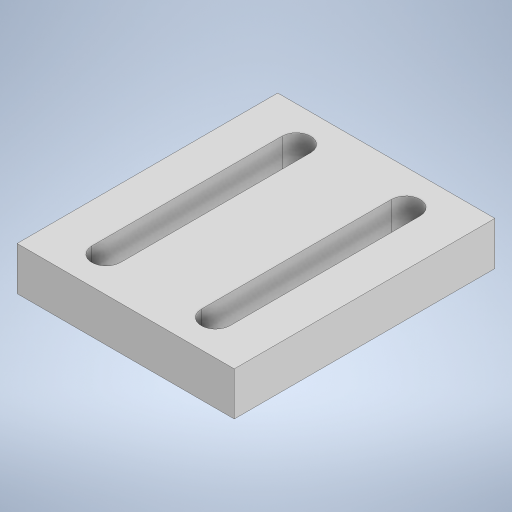
# Autodesk Inventor part: Fuß Steher
Saved by Autodesk Inventor 2024 (Build 280153000, 153)
## iProperties
Created: 2024-03-08
Part Number: Fuß Steher
Material: Generisch
Document SubType Name: Modeling
Designer: Andreas Weber
Density: 1 g/cm^3
Appearance: Vorgabe
Author: Andreas Weber
Autodesk Inventor part; units mm, degrees
ref_plane "YZ Plane" through (0, 0, 0) normal (1, 0, 0) x (0, 1, 0)
ref_plane "XZ Plane" through (0, 0, 0) normal (0, 1, 0) x (-1, 0, 0)
ref_plane "XY Plane" through (0, 0, 0) normal (0, 0, 1) x (1, 0, 0)
sketch "Skizze3" plane through (0, 0, 0) normal (0, 0, 1) x (1, 0, 0)
  line L0 (0, 0) -> (50, 0)
  line L1 (0, 0) -> (50, 0)
  line L2 (50, 0) -> (50, -60)
  line L3 (50, -60) -> (0, -60)
  line L4 (0, -60) -> (0, 0)
  line L5 (40.9, -4.8) -> (34.3, -4.8)
  line L6 (34.3, -4.8) -> (34.3, -55.2)
  line L7 (34.3, -55.2) -> (40.9, -55.2)
  line L8 (40.9, -55.2) -> (40.9, -4.8)
  line L9 (9.1, -4.8) -> (15.7, -4.8)
  line L10 (15.7, -4.8) -> (15.7, -55.2)
  line L11 (15.7, -55.2) -> (9.1, -55.2)
  line L12 (9.1, -55.2) -> (9.1, -4.8)
  dimension "d20" = 50
  dimension "d21" = 60
  dimension "d27" = 6.6
  dimension "d28" = 6.6
  constraints: 26 end point, 6 parallel, 4 horizontal, 3 perpendicular, 1 point on line
  measures "d20" distance of L2.end L3.end
  measures "d21" distance of L1.end L2.end
  measures "d27" distance of L7.end L6.end
  measures "d28" distance of L10.end L11.end
extrude "Extrusion6" add sketch "Skizze3" along normal blind 10
fillet "Rundung5" radius 3.3 8 edges at (34.3, -4.8, 5) (9.1, -4.8, 5) (40.9, -4.8, 5) (15.7, -4.8, 5) (34.3, -55.2, 5) (9.1, -55.2, 5) (40.9, -55.2, 5) (15.7, -55.2, 5)
